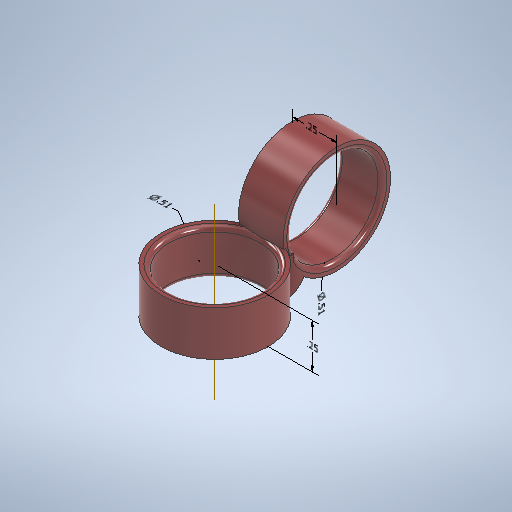
# Autodesk Inventor part: dowel-dowel
Saved by Autodesk Inventor 2025.2 (Build 292293000, 293)
## iProperties
Created: 2025-04-18
Part Number: dowel-dowel
Material: Generic
Document SubType Name: Modeling
Designer: 3lin2
Density: 1 g/cm^3
Appearance: Default
Author: 3lin2
Autodesk Inventor part; units mm, degrees
ref_plane "YZ Plane" through (0, 0, 0) normal (1, 0, 0) x (0, 1, 0)
ref_plane "XZ Plane" through (0, 0, 0) normal (0, 1, 0) x (-1, 0, 0)
ref_plane "XY Plane" through (0, 0, 0) normal (0, 0, 1) x (1, 0, 0)
sketch "Sketch2" plane through (0, 0, 0) normal (0, 1, 0) x (-1, 0, 0)
  circle A0 centre (0, 0) radius 6.477
  circle A1 centre (0, 0) radius 7.62
  dimension "d2" = 12.954
  dimension "d3" = 15.24
  constraints: 2 centre point, 2 coincident
  measures "d2" diameter of A0
  measures "d3" diameter of A1
extrude "Extrusion1" add sketch "Sketch2" along normal blind 6.35
sketch "Sketch5" plane through (0, 6.35, 0) normal (0, 1, 0) x (1, 0, 0)
  line L0 (-7.62, -7.62) -> (7.62, -7.62)
  line L1 (7.62, -7.62) -> (7.62, 7.62)
  line L2 (7.62, 7.62) -> (-7.62, 7.62)
  line L3 (-7.62, 7.62) -> (-7.62, -7.62)
  point P0 (0, 0)
  dimension "d7" = 15.24
  dimension "d8" = 15.24
  dimension "d9" = 7.62
  dimension "d10" = 7.62
  constraints: 8 end point, 2 parallel, 1 horizontal, 1 perpendicular
  measures "d7" distance of L2.end L1.end
  measures "d8" distance of L1.end L0.end
  measures "d9" distance from line of point (0, 0) L2
  measures "d10" distance from line of L1 point (0, 0)
ref_plane "Work Plane4" through (0, 6.35, -7.62) normal (0, 0, -1) x (-1, 0, 0)
ref_plane "Work Plane3" through (0, 6.35, 0) normal (0, 0, -1) x (-1, 0, 0)
ref_plane "Work Plane5" through (0, 0, 0) normal (-1, 0, 0) x (0, 1, 0)
sketch "Sketch8" plane through (0, 0, 0) normal (-1, 0, 0) x (0, 1, 0)
  circle A0 centre (7.62, 14.1945) radius 6.477
  circle A1 centre (7.62, 14.1945) radius 7.62
  line L0 (0, -7.62) -> (0, 7.62) projected
  point P0 (0, 0)
  dimension "d13" = 12.954
  dimension "d14" = 15.24
  dimension "d15" = 7.62
  constraints: 2 centre point, 1 coincident
  measures "d13" diameter of A0
  measures "d14" diameter of A1
  measures "d15" distance from line of L0 A0.centre
extrude "Extrusion2" add sketch "Sketch8" along normal mid plane 6.35
sketch "Sketch10" plane through (0, 6.35, -7.62) normal (0, 0, -1) x (-1, 0, 0)
  line L0 (-6.477, -6.35) -> (6.477, -6.35) projected
  line L1 (3.175, 7.747) -> (3.175, -5.207) projected
  line L2 (-3.175, -6.35) -> (3.175, -6.35)
  line L3 (3.175, -6.35) -> (3.175, -3.235)
  line L4 (3.175, -3.235) -> (-3.175, -3.235)
  line L5 (-3.175, -3.235) -> (-3.175, -6.35)
  line L6 (-3.175, 8.89) -> (-3.175, -6.35) projected
  point P0 (0, -6.35)
  point P1 (-3.175, -1.0208)
  point P2 (-3.175, 0)
  dimension "d28" = 0
  constraints: 8 end point, 2 parallel, 2 point on line, 1 horizontal, 1 perpendicular
  measures "d28" distance between parallel lines of L6 L5
extrude "Extrusion3" add sketch "Sketch10" along normal blind 1.8796 and the other way blind 0.9398
fillet "Fillet1" radius 3.175 1 edges at (0, 0, -9.4996)
fillet "Fillet3" radius 0.635 2 edges at (6.477, 0, 0) (6.477, 6.35, 0)
fillet "Fillet4" radius 0.635 2 edges at (-3.175, 1.143, -14.1945) (3.175, 1.143, -14.1945)
sketch "Sketch13" plane through (-3.175, 3.115, -8.0489) normal (0, 1, 0) x (1, 0, 0)
  line L0 (0, 0) -> (6.35, 0) projected
  line L1 (0, 0) -> (6.35, 0)
  line L2 (6.35, 0) -> (6.35, -1.1218)
  line L3 (0, -0.5965) -> (0, 0)
  arc A0 (6.35, -1.1218) -> (0, -1.1218) centre (3.175, -8.0489) ccw projected
  line L4 (0, -1.1218) -> (6.35, -1.1218)
  line L5 (6.35, -1.1218) -> (6.35, 0)
  line L6 (6.35, 0) -> (0, 0)
  line L7 (0, 0) -> (0, -1.1218)
  point P0 (3.175, -8.0489)
  constraints: 14 end point, 3 parallel, 2 horizontal, 2 perpendicular
extrude "Extrusion5" add sketch "Sketch13" along normal blind 2.032 contours L0 L2 A0 L7 L3
body "Solid1"
